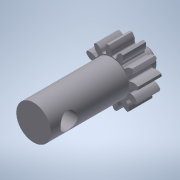
# Autodesk Inventor part: gear
Saved by Autodesk Inventor 2020 (Build 240168000, 168)
## iProperties
Created: 2003-01-31
Part Number: gear
Document SubType Name: Modeling
Designer: bhandley
Density: 1 g/cm^3
Material: Generic
Appearance: Aluminum - Flat
Control State: 0
Master: False
Checked Out: False
Shininess: 64.0
Angle Display Precision: 2
Document Length Units: 11272
Document Angle Units: 11279
Document Time Units: 11290
Document Mass Units: 11286
Document Length Units Precision: 3
Document Angle Units Precision: 2
Density: 0.0
Volumn: 0.0
Area: 0.0
PropertySet Name: Model Information
Author: bhandley
Autodesk Inventor part; units mm, degrees
ref_plane "YZ Plane" through (0, 0, 0) normal (1, 0, 0) x (0, 1, 0)
sketch "Sketch1" plane through (0, 0, 0) normal (0, 0, 1) x (1, 0, 0)
  circle A0 centre (0, 0) radius 12.7
  circle A1 centre (0, 0) radius 10.0533
  dimension "d0" = 25.4
  dimension "d1" = 2.6467
  constraints: 2 centre point, 1 coincident
  measures "d0" diameter of A0
  measures "d1" radial gap between concentric circles of A1 A0
extrude "Extrusion1" add sketch "Sketch1" along normal blind 12.7 contours A1
sketch "Sketch2" plane through (0, 0, 12.7) normal (0, 0, 1) x (1, 0, 0)
  arc A0 (14.7407, 1.4905) -> (14.6588, 2.1515) centre (0, 0) ccw
  circle A1 centre (0, 0) radius 12.7
  circle A2 centre (0, 0) radius 11.9342
  line L0 (10.0533, 0) -> (11.9342, 0)
  spline S0 degree 4 poles (11.9342, 0) (12.0401, -0.0103) (12.8324, 0.1732) (13.5154, 0.4752) (14.7274, 1.4614) (14.7407, 1.4905) knots 0 0 0 0 0 0.456983 1 1 1 1 1
  circle A3 centre (12.6986, 0.1882) radius 3.3147
  line L1 (14.6588, 2.1515) -> (9.9468, 1.4599)
  arc A4 (10.0533, 0) -> (9.9468, 1.4599) centre (0, 0) ccw
  line L2 (10.0533, 0) -> (11.9342, 0)
  point P0 (12.6416, 0.1676)
  point P1 (13.4595, 0.5563)
  point P2 (14.5009, 1.2878)
  dimension "d4" = 25.4
  dimension "d6" = 23.8684
  dimension "d5" = 2.1158
  dimension "d7" = 12.1158
  dimension "d8" = 0.0203
  dimension "d9" = 12.6416
  dimension "d10" = 0.1676
  dimension "d11" = 13.4595
  dimension "d12" = 0.5563
  dimension "d13" = 14.5009
  dimension "d14" = 1.2878
  dimension "d17" = 6.6294
  constraints: 6 end point, 5 coincident, 4 point on circle, 3 centre point, 1 collinear, 1 horizontal, 14 other
  measures "d7" distance of point (0, 0) point (12.116, 0.02)
  measures "d8" vertical distance of point (0, 0) point (12.116, 0.02)
  measures "d9" horizontal distance of point (0, 0) point (12.642, 0.168)
  measures "d10" vertical distance of point (0, 0) point (12.642, 0.168)
  measures "d11" horizontal distance of point (0, 0) point (13.459, 0.556)
  measures "d12" vertical distance of point (0, 0) point (13.459, 0.556)
  measures "d13" horizontal distance of point (0, 0) point (14.501, 1.288)
  measures "d14" vertical distance of point (0, 0) point (14.501, 1.288)
  measures "d17" diameter of A3
extrude "Extrusion2" add sketch "Sketch2" against normal blind 12.7 contours S0 A1 L1 A0 | S0 A2 L1 A1 | L0 A4 L1 A2
mirror "Mirror1" about plane through (14.6588, 2.1515, 12.7) normal (-0.1452183, 0.9893996, 0) of "Extrusion2"
fillet "Fillet1" radius 0.7976 2 edges at (9.6293, 2.8889, 6.35) (10.0533, 0, 6.35)
pattern_circular "Circular Pattern1" count 12 over 360 about axis through (0, 0, 0) along (0, 0, 1) of "Extrusion2", "Mirror1", "Fillet1"
ref_plane "Work Plane2" through (0, 0, 0) normal (1, 0, 0) x (0, 1, 0)
ref_plane "Work Plane3" through (0, 0, 0) normal (1, 0, 0) x (0, 0, 1)
sketch "Sketch9" plane through (0, 0, 12.7) normal (0, 0, 1) x (1, 0, 0)
  circle A0 centre (0, 0) radius 9.506
  dimension "d60" = 19.0119
  constraints: 1 centre point, 1 coincident
  measures "d60" diameter of A0
extrude "Extrusion6" add sketch "Sketch9" along normal blind 42.8498
sketch "Sketch10" plane through (0, 0, 0) normal (1, 0, 0) x (0, 1, 0)
  circle A0 centre (0, 45.5168) radius 4.7625
  line L0 (9.506, 55.5498) -> (-9.506, 55.5498) projected
  point P0 (0, 0)
  point P1 (0, 55.5498)
  dimension "d63" = 9.525
  dimension "d64" = 10.033
  constraints: 1 centre point, 1 midpoint, 1 vertical alignment
  measures "d63" diameter of A0
  measures "d64" distance from line of A0.centre L0
extrude "Extrusion7" cut sketch "Sketch10" along normal through all both and the other way through all
sketch "Sketch11" plane through (0, 0, 0) normal (0, 0, -1) x (-1, 0, 0)
  circle A0 centre (0, 0) radius 6.2547
  dimension "d67" = 12.5095
  constraints: 1 centre point, 1 coincident
  measures "d67" diameter of A0
extrude "Extrusion8" add sketch "Sketch11" along normal blind 6.35
chamfer "Chamfer2" distance 0.762 angle 45 1 edges at (6.2547, 0, -6.35)
sketch "Sketch12" plane through (0, 0, -6.35) normal (0, 0, -1) x (-1, 0, 0)
  point P0 (0, 0)
  point P1 (0, 0)
  constraints: 1 coincident
hole "Hole4" at (0, 0, -6.35) direction (0, 0, 1) diameter 4.9784 depth 10.16 tip angle 118 thread size "1/4-20 UNC" class "2B" standard "ANSI Unified Screw Threads"
body "Solid1"
